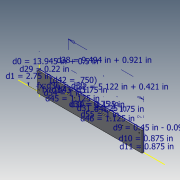
# Autodesk Inventor part: VP SWITCHMNT B
Saved by Autodesk Inventor 2018.3 (Build 223284000, 284)
## iProperties
Created: 2020-01-27
Material: Generic
Vendor: HHMI: JRC - ID&F
Document SubType Name: Modeling
Designer: arnoldj
Density: 1 g/cm^3
Appearance: Default
RuleStatus: InUse
AfterDocSave0: file://Part Number Cleaner
DESIGN DEPARTMENT: HHMI: JRC - ID&F
ALTERED ITEM PART NUMBER: N/A
ALTERED ITEM VENDOR: N/A
ALTERED ITEM DESCRIPTION: N/A
Author: arnoldj
Revision Number: 0
Autodesk Inventor part; units mm, degrees
ref_plane "YZ Plane" through (0, 0, 0) normal (1, 0, 0) x (0, 1, 0)
ref_plane "XZ Plane" through (0, 0, 0) normal (0, 1, 0) x (-1, 0, 0)
sketch "Sketch1" plane through (0, 0, 0) normal (0, 0, 1) x (1, 0, 0)
  line L0 (0, 83.82) -> (0, -13.97) projected
  line L1 (-73.3806, 0) -> (440.2836, 0) projected
  line L2 (0, 0) -> (366.903, 0)
  line L3 (366.903, 0) -> (366.903, 69.85)
  line L4 (366.903, 69.85) -> (0, 69.85)
  line L5 (0, 69.85) -> (0, 0)
  line L6 (0, 34.925) -> (366.903, 34.925) construction
  line L7 (241.9858, 50.8) -> (210.2358, 50.8) construction
  line L8 (241.9858, 52.3875) -> (210.2358, 52.3875)
  line L9 (210.2358, 49.2125) -> (241.9858, 49.2125)
  arc A0 (241.9858, 49.2125) -> (241.9858, 52.3875) centre (241.9858, 50.8) ccw
  arc A1 (210.2358, 52.3875) -> (210.2358, 49.2125) centre (210.2358, 50.8) ccw
  line L10 (118.237, 50.8) -> (86.487, 50.8) construction
  line L11 (118.237, 52.3875) -> (86.487, 52.3875)
  line L12 (86.487, 49.2125) -> (118.237, 49.2125)
  arc A2 (118.237, 49.2125) -> (118.237, 52.3875) centre (118.237, 50.8) ccw
  arc A3 (86.487, 52.3875) -> (86.487, 49.2125) centre (86.487, 50.8) ccw
  line L13 (102.362, 50.8) -> (366.903, 50.8) construction
  point P0 (5.588, 12.7)
  point P1 (5.588, 57.15)
  point P2 (357.7717, 57.15)
  point P3 (357.7717, 12.7)
  point P4 (226.1108, 50.8)
  point P5 (226.1108, 50.8)
  point P6 (130.937, 50.8)
  point P7 (299.1358, 50.8)
  point P8 (254.6858, 50.8)
  point P9 (175.387, 50.8)
  point P10 (76.962, 50.8)
  point P11 (200.7108, 50.8)
  dimension "d0" = 366.903
  dimension "d1" = 69.85
  dimension "d9" = 9.1313
  dimension "d10" = 22.225
  dimension "d11" = 22.225
  dimension "d29" = 5.588
  dimension "d30" = 3.175
  dimension "d31" = 31.75
  dimension "d32" = 140.7922
  dimension "d33" = 19.05
  dimension "d36" = 3.175
  dimension "d37" = 31.75
  dimension "d38" = 264.541
  dimension "d41" = 44.45
  dimension "d42" = 19.05
  dimension "d43" = 44.45
  dimension "d45" = 28.575
  dimension "d46" = 28.575
  dimension "d54" = 25.4
  dimension "d55" = 25.4
  constraints: 28 end point, 8 point on circle, 8 tangent, 7 point on line, 4 centre point, 4 midpoint, 4 parallel, 3 horizontal, 2 coincident, 2 horizontal alignment, 2 vertical alignment, 1 perpendicular
  measures "d0" distance of L3.end L4.end
  measures "d1" distance of L4.end L2.start
  measures "d9" distance from line of point (357.772, 57.15) L3
  measures "d10" distance from line of point (357.772, 57.15) L6
  measures "d11" distance from line of L6 point (357.772, 12.7)
  measures "d29" distance from line of point (5.588, 57.15) L0
  measures "d30" distance between parallel lines of L8 L9
  measures "d31" distance of L8.start L8.end
  measures "d32" distance from line of L3 point (226.111, 50.8)
  measures "d33" distance between parallel lines of L4 L7
  measures "d36" distance between parallel lines of L11 L12
  measures "d37" distance of L11.start L11.end
  measures "d38" distance from line of L3 L13.start
  measures "d41" distance of point (254.686, 50.8) point (299.136, 50.8)
  measures "d42" distance between parallel lines of L4 L13
  measures "d43" distance of point (130.937, 50.8) point (175.387, 50.8)
  measures "d45" distance of point (130.937, 50.8) L13.start
  measures "d46" distance of point (254.686, 50.8) point (226.111, 50.8)
  measures "d54" distance of point (76.962, 50.8) point (102.362, 50.8)
  measures "d55" distance of point (226.111, 50.8) point (200.711, 50.8)
extrude "Extrusion1" add sketch "Sketch1" along normal blind 5.842 contours L4 L3 L1 L0 | A0 L9 A1 L8 | A2 L12 A3 L11
hole "Hole1" at (357.7717, 57.15, 0) at (357.7717, 12.7, 0) direction (0, 0, 1) diameter 3.81 end through all
hole "Hole2" at (5.588, 12.7, 0) at (5.588, 57.15, 0) direction (0, 0, 1) diameter 3.81 end through all
extrude "Extrusion2" cut sketch "Sketch1" along normal up to next contours A0 L9 A1 L8 | A2 L12 A3 L11
hole "Hole3" at (130.937, 50.8, 0) at (299.1358, 50.8, 0) at (254.6858, 50.8, 0) at (76.962, 50.8, 0) at (200.7108, 50.8, 0) direction (0, 0, 1) diameter 2.3622 end through all
equation "\"d36\" = d30"
equation "\"d37\" = d31"
body "Solid1"
